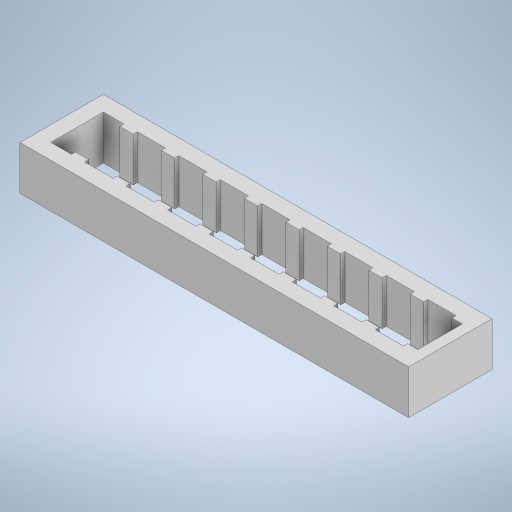
# Autodesk Inventor part: LatchHolder
Saved by Autodesk Inventor 2024 (Build 280153000, 153)
## iProperties
Created: 2024-03-21
Part Number: LatchHolder
Material: Generic
Document SubType Name: Modeling
Designer: gcter
Density: 1 g/cm^3
Appearance: Default
Author: gcter
Autodesk Inventor part; units mm, degrees
ref_plane "YZ Plane" through (0, 0, 0) normal (1, 0, 0) x (0, 1, 0)
ref_plane "XZ Plane" through (0, 0, 0) normal (0, 1, 0) x (-1, 0, 0)
ref_plane "XY Plane" through (0, 0, 0) normal (0, 0, 1) x (1, 0, 0)
sketch "Sketch1" plane through (0, 0, 0) normal (0, 1, 0) x (-1, 0, 0)
  line L0 (0, 0) -> (0, -20.574)
  line L1 (0, -20.574) -> (-8.89, -20.574)
  line L2 (-8.89, -20.574) -> (-8.89, -16.764)
  line L3 (-8.89, -16.764) -> (-3.81, -16.764)
  line L4 (-3.81, -16.764) -> (-3.81, -3.81)
  line L5 (-3.81, -3.81) -> (-8.89, -3.81)
  line L6 (-8.89, -3.81) -> (-8.89, 0)
  line L7 (-8.89, 0) -> (0, 0)
  point P0 (0, -10.287)
  dimension "d1" = 20.574
  dimension "d2" = 3.81
  dimension "d3" = 3.81
  dimension "d4" = 3.81
  dimension "d5" = 5.08
  constraints: 16 end point, 7 perpendicular, 1 collinear, 1 midpoint, 1 vertical
  measures "d1" distance between parallel lines of L7 L1
  measures "d2" distance between parallel lines of L3 L1
  measures "d3" distance between parallel lines of L7 L5
  measures "d4" distance from line of L4 point (0, -10.287)
  measures "d5" distance between parallel lines of L4 L2
extrude "Extrusion1" add sketch "Sketch1" along normal blind 10.8712
sketch "Sketch2" plane through (0, 0, 0) normal (0, -1, 0) x (1, 0, 0)
  line L0 (8.89, -20.574) -> (8.89, -15.748)
  line L1 (8.89, -15.748) -> (12.192, -15.748)
  line L2 (12.192, -15.748) -> (12.192, -16.764)
  line L3 (12.192, -16.764) -> (19.1262, -16.764)
  line L4 (19.1262, -16.764) -> (19.1262, -20.574)
  line L5 (19.1262, -20.574) -> (8.89, -20.574)
  line L6 (3.81, -16.764) -> (8.89, -16.764) projected
  line L7 (8.89, 0) -> (8.89, -3.81) projected
  line L8 (8.89, 0) -> (8.89, -4.826)
  line L9 (8.89, -4.826) -> (12.192, -4.826)
  line L10 (12.192, -4.826) -> (12.192, -3.81)
  line L11 (12.192, -3.81) -> (19.1262, -3.81)
  line L12 (19.1262, -3.81) -> (19.1262, 0)
  line L13 (0, 0) -> (8.89, 0) projected
  line L14 (19.1262, 0) -> (8.89, 0)
  line L15 (8.89, -3.81) -> (3.81, -3.81) projected
  dimension "d8" = 3.302
  dimension "d9" = 6.9342
  dimension "d10" = 1.016
  dimension "d11" = 1.016
  constraints: 24 end point, 9 perpendicular, 6 collinear, 1 vertical
  measures "d8" distance between parallel lines of L0 L2
  measures "d9" distance between parallel lines of L4 L2
  measures "d10" distance between parallel lines of L1 L3
  measures "d11" distance between parallel lines of L15 L9
extrude "Extrusion2" add sketch "Sketch2" against normal up to surface (10.8712 mm away)
pattern_linear "Rectangular Pattern1" count 8 spacing 10.2362 along (1, 0, 0) of "Extrusion2"
sketch "Sketch3" plane through (0, 0, 0) normal (0, -1, 0) x (1, 0, 0)
  line L0 (0, -20.574) -> (90.7796, -20.574) projected
  line L1 (90.7796, -20.574) -> (90.7796, -15.748)
  line L2 (90.7796, -20.574) -> (90.7796, -16.764) projected
  line L3 (90.7796, -15.748) -> (93.3196, -15.748)
  line L4 (93.3196, -15.748) -> (93.3196, -4.826)
  line L5 (93.3196, -4.826) -> (90.7796, -4.826)
  line L6 (90.7796, -4.826) -> (90.7796, 0)
  line L7 (90.7796, 0) -> (95.8596, 0)
  line L8 (95.8596, 0) -> (95.8596, -20.574)
  line L9 (95.8596, -20.574) -> (90.7796, -20.574)
  line L10 (83.8454, -15.748) -> (80.5434, -15.748) projected
  line L11 (80.5434, -4.826) -> (83.8454, -4.826) projected
  line L12 (90.7796, 0) -> (0, 0) projected
  dimension "d17" = 5.08
  dimension "d18" = 2.54
  constraints: 16 end point, 6 perpendicular, 4 collinear, 2 point on line
  measures "d17" distance between parallel lines of L1 L8
  measures "d18" distance between parallel lines of L1 L4
extrude "Extrusion3" add sketch "Sketch3" against normal up to surface (10.8712 mm away)
body "Solid1"
